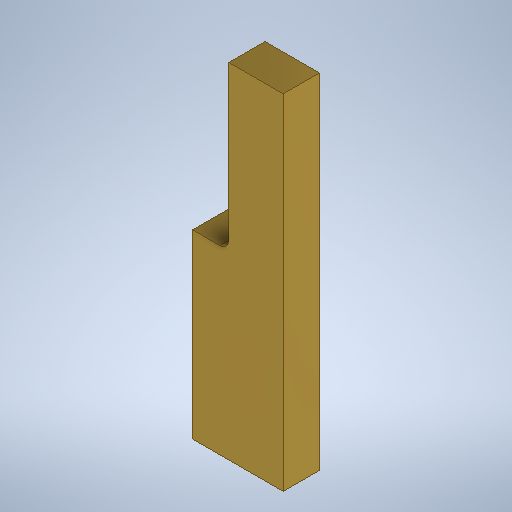
# Autodesk Inventor part: pins
Saved by Autodesk Inventor 2025 (Build 290162000, 162)
## iProperties
Created: 2025-09-08
Part Number: pins
Material: Gold
Document SubType Name: Modeling
Designer: jirne
Density: 19.3 g/cm^3
Appearance: Metal 1600F Hot
Author: jirne
Autodesk Inventor part; units mm, degrees
ref_plane "YZ Plane" through (0, 0, 0) normal (1, 0, 0) x (0, 1, 0)
ref_plane "XZ Plane" through (0, 0, 0) normal (0, 1, 0) x (-1, 0, 0)
ref_plane "XY Plane" through (0, 0, 0) normal (0, 0, 1) x (1, 0, 0)
sketch "Sketch1" plane through (0, 0, 0) normal (0, 1, 0) x (-1, 0, 0)
  line L0 (0, 0) -> (-0.762, 0)
  line L1 (-0.762, 0) -> (-0.762, 2.286)
  line L2 (-0.762, 2.286) -> (0, 2.286)
  line L3 (0, 2.286) -> (0, 0)
  dimension "d0" = 0.762
  dimension "d1" = 2.286
  constraints: 8 end point, 2 parallel, 1 horizontal, 1 perpendicular
  measures "d0" distance of L1.end L2.end
  measures "d1" distance of L0.end L1.end
extrude "Extrusion1" add sketch "Sketch1" along normal blind 0.508
sketch "Sketch2" plane through (0.762, 0, 0) normal (0, 0, -1) x (-1, 0, 0)
  line L0 (0.762, 0) -> (0, 0) projected
  line L1 (0, 0) -> (1.27, 0)
  line L2 (1.27, 0) -> (1.27, 0.508)
  line L3 (1.27, 0.508) -> (0, 0.508)
  line L4 (0, 0.508) -> (0, 0)
  dimension "d4" = 1.27
  constraints: 8 end point, 2 parallel, 1 horizontal, 1 perpendicular
  measures "d4" distance of L0.end L1.end
extrude "Extrusion2" add sketch "Sketch2" along normal blind 2.54
fillet "Fillet1" radius 0.127 1 edges at (0, 0.254, 0)
body "Solid1"
